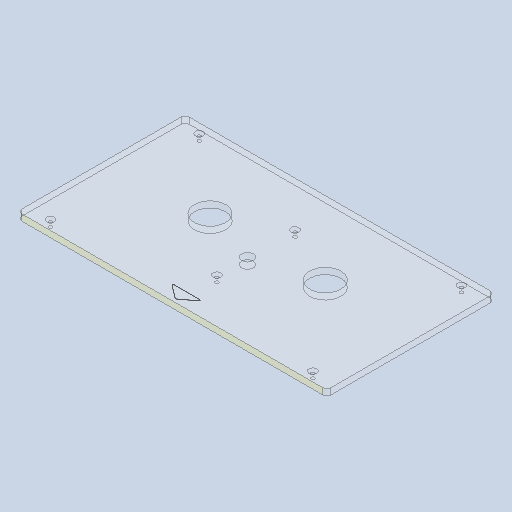
# Autodesk Inventor part: Base Pressor 1
Saved by Autodesk Inventor 2026 (Build 300175050, 175E)
## iProperties
Company: Delta
Created: 2025-08-15
Part Number: Base Pressor 1
Material: Acrílico TP
Document SubType Name: Modeling
Density: 1.19 g/cm^3
Appearance: Transparente - Claro
Project: FCT
Description: Base Pressor 1
Mass: 948.25 g
Surface Area: 1735.03 cm^2
Volume: 796.849 cm^3
Checked By: William Pinheiro
Engr Approved By: Antonio Lucas
Acabamento: N/A
Dimensões: 10 x 214 x 375
Total: 1
Author: Kedson Neves
Revision Number: 01
Title: FCT
Autodesk Inventor part; units mm, degrees
ref_plane "YZ Plane" through (0, 0, 0) normal (1, 0, 0) x (0, 1, 0)
ref_plane "XZ Plane" through (0, 0, 0) normal (0, 1, 0) x (-1, 0, 0)
ref_plane "XY Plane" through (0, 0, 0) normal (0, 0, 1) x (1, 0, 0)
sketch "Sketch1" plane through (0, 0, 0) normal (0, 0, 1) x (1, 0, 0)
  line L0 (-262.5, 0) -> (262.5, 0) construction
  line L1 (0, -149.8) -> (0, 149.8) construction
  line L2 (-187.5, 107) -> (187.5, 107)
  line L3 (187.5, 107) -> (187.5, -107)
  line L4 (187.5, -107) -> (-187.5, -107)
  line L5 (-187.5, -107) -> (-187.5, 107)
  point P0 (-167.5, 95)
  point P1 (167.5, 95)
  point P2 (-167.5, -95)
  point P3 (167.5, -95)
  point P4 (0, 0)
  point P5 (-175, 0)
  point P6 (175, 0)
  point P7 (0, -50)
  point P8 (0, 50)
  point P9 (0, 20)
  point P10 (175, 20)
  point P11 (-175, 20)
  dimension "d0" = 375
  dimension "d1" = 214
  dimension "d3" = 335
  dimension "d30" = 20
  dimension "d45" = 12
  dimension "d46" = 190
  dimension "d47" = 100
  dimension "d48" = 12.5
  dimension "d52" = 20
  constraints: 8 end point, 6 symmetric about line, 5 point on line, 2 horizontal alignment, 2 midpoint, 2 parallel, 1 horizontal, 1 perpendicular, 1 vertical alignment, 2 other
  measures "d0" distance between parallel lines of L3 L5
  measures "d1" distance between parallel lines of L4 L2
  measures "d3" distance of point (167.5, 95) point (-167.5, 95)
  measures "d30" distance from line of L5 point (-167.5, 95)
  measures "d45" distance from line of L2 point (-167.5, 95)
  measures "d46" distance of point (-167.5, -95) point (-167.5, 95)
  measures "d47" distance of point (0, -50) point (0, 50)
  measures "d48" distance from line of L5 point (-175, 0)
  measures "d52" distance of point (-175, 20) point (-175, 0)
extrude "Extrusion1" add sketch "Sketch1" against normal blind 8
hole "Hole1" at (-167.5, 95, 0) at (167.5, 95, 0) at (-167.5, -95, 0) at (167.5, -95, 0) at (0, -50, 0) at (0, 50, 0) direction (0, 0, -1) diameter 4.5 end through all countersink diameter 10 countersink angle 90 clearance for "Countersunk Flat Head Hex Socket Screw ISO 10642" size "M4" standard "ISO"
hole "Hole2" at (0, 0, 0) at (0, 20, 0) direction (0, 0, -1) diameter 10.647 end through all thread size "M12x1.25" class "6H" standard "ISO Metric profile"
sketch "Sketch2" plane through (0, 0, -8) normal (0, 0, -1) x (-1, 0, 0)
  point P0 (0, 0)
  point P1 (175, 0)
  point P2 (175, 0)
  point P3 (-175, 0)
  point P4 (-175, 0)
  point P5 (0, 20)
  point P6 (0, 0)
  point P7 (175, 20)
  point P8 (-175, 20)
  constraints: 2 coincident
hole "Hole4" at (-175, 0, -8) at (175, 0, -8) at (-175, 20, -8) at (175, 20, -8) direction (0, 0, 1) diameter 6.5 end through all countersink diameter 14.5 countersink angle 90 clearance for "Countersunk Flat Head Hex Socket Screw ISO 10642" size "M6" standard "ISO"
fillet "Arredondamento2" radius 5 4 edges at (187.5, -107, -4) (187.5, 107, -4) (-187.5, -107, -4) (-187.5, 107, -4)
sketch "Esboço3" plane through (0, 0, 0) normal (0, 0, 1) x (1, 0, 0)
  line L0 (0, -149.8) -> (0, 149.8) construction
  line L1 (-262.5, 0) -> (262.5, 0) construction
  line L2 (-182.5, -107) -> (182.5, -107) construction
  line L3 (-17.12, -90.16) -> (-0.72, -102.46)
  line L4 (17.12, -90.16) -> (0.72, -102.46)
  line L5 (-16.4, -88) -> (16.4, -88)
  line L6 (17, -90) -> (0.6, -102.3)
  line L7 (-0.6, -102.3) -> (-17, -90)
  line L8 (-16.4, -88.2) -> (16.4, -88.2)
  arc A0 (-16.4, -88) -> (-17.12, -90.16) centre (-16.4, -89.2) ccw
  arc A1 (17.12, -90.16) -> (16.4, -88) centre (16.4, -89.2) ccw
  arc A2 (-0.72, -102.46) -> (0.72, -102.46) centre (0, -101.5) ccw
  arc A3 (-16.4, -88.2) -> (-17, -90) centre (-16.4, -89.2) ccw
  arc A4 (17, -90) -> (16.4, -88.2) centre (16.4, -89.2) ccw
  arc A5 (-0.6, -102.3) -> (0.6, -102.3) centre (0, -101.5) ccw
  point P0 (0, 0)
  point P1 (0, -103)
  point P2 (20, -88)
  point P3 (-20, -88)
  point P4 (19.4, -88.2)
  point P5 (0, -102.75)
  point P6 (-19.4, -88.2)
  dimension "d53" = 40
  dimension "d54" = 15
  dimension "d55" = 0.2
  dimension "d56" = 4
  dimension "d59" = 1.2
  dimension "d60" = 1
  constraints: 12 end point, 12 point on circle, 12 point on line, 12 tangent, 6 centre point, 4 equal radius, 1 horizontal, 3 other
  measures "d53" distance of point (-20, -88) point (20, -88)
  measures "d54" distance from line of L5 point (0, -103)
  measures "d55" distance between parallel lines of L5 L8
  measures "d56" distance from line of L2 point (0, -103)
  measures "d59" radius of A0
  measures "d60" radius of A3
emboss "Relevo1" sketch "Esboço3" operation cut depth 0.1 direction (0, 0, -1)
move faces "Mover1" translate (10, 0, 0) faces at (187.5, -34, -2.6667) (183.2452, -106.9442, -2.6667) (187.4442, 102.7452, -2.6667)
move faces "Mover2" translate (-10, 0, 0) faces at (-187.5, 34, -2.6667)
sketch "Esboço4" plane through (0, 0, 0) normal (0, 0, 1) x (1, 0, 0)
  line L0 (197.5, -96.337) -> (195.5, -98.337) construction
  line L1 (197.5, -96.337) -> (197.5, 74.663) construction
  line L2 (195.5, 76.663) -> (197.5, 74.663) construction
  line L3 (195.5, 76.663) -> (-195.5, 76.663) construction
  line L4 (-197.5, 74.663) -> (-195.5, 76.663) construction
  line L5 (-197.5, 74.663) -> (-197.5, -96.337) construction
  line L6 (-195.5, -98.337) -> (-197.5, -96.337) construction
  line L7 (-195.5, -98.337) -> (195.5, -98.337) construction
  circle A0 centre (175, -10.837) radius 10 construction
  circle A1 centre (-175, -10.837) radius 10 construction
  circle A2 centre (0, -10.837) radius 5.3235 construction
  circle A3 centre (0, -10.837) radius 7.5286
  point P0 (0, 0)
  constraints: 1 centre point, 1 coincident
extrude "Extrusão4" cut sketch "Esboço4" against normal through all
sketch "Esboço5" plane through (0, 0, 0) normal (0, 0, 1) x (1, 0, 0)
  line L0 (-13.7648, 30.5285) -> (13.2237, 30.5285)
  line L1 (13.2237, 30.5285) -> (13.2237, -4.2725)
  line L2 (13.2237, -4.2725) -> (-13.7648, -4.2725)
  line L3 (-13.7648, -4.2725) -> (-13.7648, 30.5285)
  arc A0 (-3.3823, -4.111) -> (3.3823, -4.111) centre (0, -10.837) ccw projected
  circle A1 centre (0, -10.837) radius 7.5286
  point P0 (0, 0)
  point P1 (-3.686, -4.2725)
  point P2 (-3.3823, -4.111)
  point P3 (3.3823, -4.111)
  point P4 (3.686, -4.2725)
  constraints: 8 end point, 2 parallel, 1 centre point, 1 coincident, 1 horizontal, 1 perpendicular
extrude "Extrusão5" add sketch "Esboço5" against normal up to surface (8 mm away) contours L0 L1 L2 A0 A1 L3
sketch "Esboço6" plane through (0, 0, 0) normal (0, 0, 1) x (1, 0, 0)
  arc A0 (-56.8827, 0.8848) -> (-70.3997, -6.3048) centre (-72.3181, 13.603) ccw projected
  arc A1 (90.3173, 0.8848) -> (76.8003, -6.3048) centre (74.8819, 13.603) ccw projected
  circle A2 centre (-72.3181, 13.603) radius 20
  circle A3 centre (74.8819, 13.603) radius 20
  point P0 (0, 0)
  point P1 (76.8003, -6.3048)
  point P2 (90.3173, 0.8848)
  point P3 (-70.3997, -6.3048)
  point P4 (-56.8827, 0.8848)
  constraints: 2 centre point, 2 coincident, 2 concentric
extrude "Extrusão6" cut sketch "Esboço6" against normal through all
sketch "Esboço7" plane through (0, 0, 0) normal (0, 0, 1) x (1, 0, 0)
  line L0 (-188.8896, -14.5971) -> (-157.1436, -14.5971)
  line L1 (-157.1436, -14.5971) -> (-157.1436, 42.0923)
  line L2 (-157.1436, 42.0923) -> (-188.8896, 42.0923)
  line L3 (-188.8896, 42.0923) -> (-188.8896, -14.5971)
  line L4 (151.9751, -26.6168) -> (188.6283, -26.6168)
  line L5 (188.6283, -26.6168) -> (188.6283, 48.0472)
  line L6 (188.6283, 48.0472) -> (151.9751, 48.0472)
  line L7 (151.9751, 48.0472) -> (151.9751, -26.6168)
  point P0 (0, 0)
  constraints: 16 end point, 4 parallel, 2 horizontal, 2 perpendicular
extrude "Extrusão7" add sketch "Esboço7" against normal up to surface (8 mm away)
equation "\"d60\" = d59 - d55"
body "Solid1"
